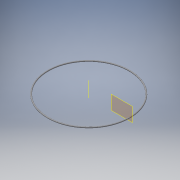
# Autodesk Inventor part: Staicring
Saved by Autodesk Inventor 2019 (Build 230136000, 136)
## iProperties
Created: 2021-01-17
Part Number: Staicring
Material: Типовые
Document SubType Name: Modeling
Designer: Dazer
Density: 1 g/cm^3
Appearance: По умолчанию
Author: Dazer
Autodesk Inventor part; units mm, degrees
ref_plane "YZ Plane" through (0, 0, 0) normal (1, 0, 0) x (0, 1, 0)
ref_plane "XZ Plane" through (0, 0, 0) normal (0, 1, 0) x (-1, 0, 0)
ref_plane "XY Plane" through (0, 0, 0) normal (0, 0, 1) x (1, 0, 0)
ref_plane "РабПлоскость1" through (0, 0, -1.5) normal (0, 0, 1) x (1, 0, 0)
sketch "Эскиз1" plane through (0, 0, -1.5) normal (0, 0, 1) x (1, 0, 0)
  circle A0 centre (22, -18.25) radius 1.25 projected
  circle A1 centre (22, -18.25) radius 1.15
  line L0 (-53, 3.9) -> (-53, -23.4) projected
  point P0 (0, 0)
  dimension "d0" = 0.1
  constraints: 1 centre point
  measures "d0" radial gap between concentric circles of A0 A1
revolve "Вращение1" add sketch "Эскиз1" angle 360 about axis through (-53, -54.25, -1.5) along (0, -1, 0) contours A1
